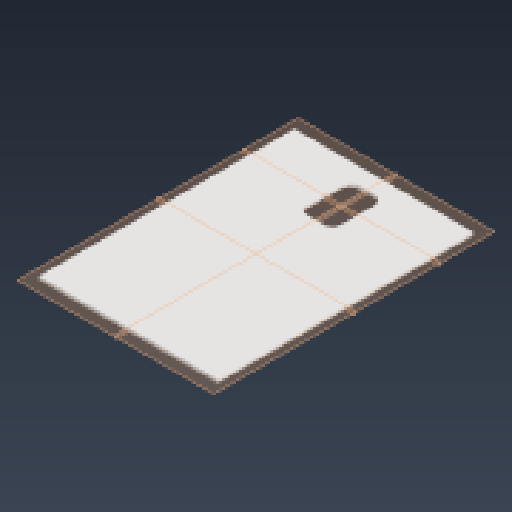
# Autodesk Inventor part: Передняя_фанера
Saved by Autodesk Inventor 2023.2 (Build 272271030, 271C)
## iProperties
Created: 2025-10-07
Part Number: Передняя_фанера
Material: Типовые
Document SubType Name: Modeling
Designer: Олег Коноваленко
Density: 1 g/cm^3
Appearance: По умолчанию
Author: Олег Коноваленко
Autodesk Inventor part; units mm, degrees
sketch "Эскиз2" plane through (0, 0, 0) normal (0, 1, 0) x (-1, 0, 0)
  line L0 (105, 150) -> (-105, 150)
  line L1 (-105, 150) -> (-105, -150)
  line L2 (-105, -150) -> (105, -150)
  line L3 (105, -150) -> (105, 150)
  line L4 (105, 150) -> (-105, -150) construction
  line L5 (-105, 150) -> (105, -150) construction
  point P0 (0, 0)
  dimension "d0" = 300
  dimension "d1" = 210
  constraints: 12 end point, 2 midpoint, 2 parallel, 1 horizontal, 1 perpendicular
  measures "d0" distance of L0.end L1.end
  measures "d1" distance of L1.end L2.end
extrude "Выдавливание1" add sketch "Эскиз2" along normal mid plane 4
sketch "Эскиз3" plane through (0, -2, 0) normal (0, -1, 0) x (1, 0, 0)
  line L0 (105, -150) -> (-105, -150) projected
  line L1 (20, -150) -> (-20, -150)
  line L2 (-20, -150) -> (-20, -70)
  line L3 (-20, -70) -> (20, -70)
  line L4 (20, -70) -> (20, -150)
  line L5 (-105, 150) -> (-105, -150) projected
  line L6 (20, -130) -> (-20, -130)
  dimension "d7" = 40
  dimension "d9" = 80
  dimension "d10" = 20
  dimension "d12" = 85
  constraints: 10 end point, 3 point on line, 2 parallel, 2 perpendicular, 1 horizontal
  measures "d7" distance of L2.end L3.end
  measures "d9" distance of L1.end L2.end
  measures "d10" distance between parallel lines of L0 L6
  measures "d12" distance between parallel lines of L5 L2
extrude "Выдавливание2" cut sketch "Эскиз3" against normal up to next contours L6 L2 L3 L4
fillet "Сопряжение1" radius 10 4 edges at (20, 0, -130) (-20, 0, -130) (-20, 0, -70) (20, 0, -70)
ref_plane "РабПлоскость1" through (-10, -2, -100) normal (0, 0, 1) x (1, 0, 0)
